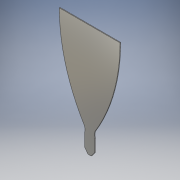
# Autodesk Inventor part: Dis
Saved by Autodesk Inventor 2018 (Build 220112000, 112)
## iProperties
Created: 2019-04-15
Part Number: Dis
Material: Generic
Document SubType Name: Modeling
Designer: This kid
Density: 1 g/cm^3
Appearance: Default
Author: This kid
Autodesk Inventor part; units mm, degrees
ref_plane "YZ Plane" through (0, 0, 0) normal (1, 0, 0) x (0, 1, 0)
ref_plane "XZ Plane" through (0, 0, 0) normal (0, 1, 0) x (-1, 0, 0)
ref_plane "XY Plane" through (0, 0, 0) normal (0, 0, 1) x (1, 0, 0)
sketch "Sketch1" plane through (0, 0, 0) normal (0, 0, 1) x (1, 0, 0)
  line L0 (-10.2957, 5.2289) -> (52.5693, 5.2289)
  line L1 (-10.2957, 5.2289) -> (15.9234, -93.8311) construction
  line L2 (15.9234, -93.8311) -> (26.3501, -93.8311) construction
  line L3 (15.9234, -93.8311) -> (15.9234, -106.5311)
  line L4 (26.3501, -93.8311) -> (26.3501, -106.5311)
  arc A0 (26.3501, -87.7106) -> (26.3501, -93.8311) centre (36.9972, -90.7709) ccw
  arc A1 (26.3501, -87.7106) -> (52.5693, 5.2289) centre (-125.2627, 5.2289) ccw
  line L5 (21.1368, 5.2289) -> (21.1368, -93.8311) construction
  arc A2 (15.9234, -93.8311) -> (15.9234, -87.7106) centre (5.2764, -90.7709) ccw
  arc A3 (-10.2957, 5.2289) -> (15.9234, -87.7106) centre (167.5363, 5.2289) ccw
  line L6 (26.3501, -106.5311) -> (23.352, -113.2427) construction
  line L7 (26.3501, -106.5311) -> (22.8287, -111.1925)
  line L8 (22.8287, -111.1925) -> (19.4449, -111.1925)
  line L9 (15.9234, -106.5311) -> (19.4449, -111.1925)
  point P0 (0, 0)
  point P1 (8.355, -65.2363)
  dimension "d10" = 10.4267
  dimension "d11" = 12.7
  dimension "d12" = 99.06
  dimension "d15" = 5.842
  dimension "d16" = 5.842
  constraints: 20 end point, 8 point on circle, 4 centre point, 3 symmetric about line, 2 point on line, 2 vertical, 1 horizontal, 1 midpoint, 1 parallel, 5 other
  measures "d10" distance of L1.end L2.end
  measures "d11" distance of L1.end L3.end
  measures "d12" vertical distance of L0.end L2.end
  measures "d15" distance of L3.end L8.end
  measures "d16" distance of L4.end L7.end
extrude "Extrusion1" add sketch "Sketch1" along normal blind 0.7112
body "Solid1"
